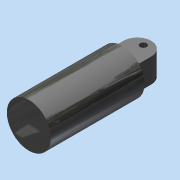
# Autodesk Inventor part: AntennaBase
Saved by Autodesk Inventor 2011 SP1 (Build 150282100, 282)
## iProperties
Created: 2011-08-14
Part Number: AntennaBase
Document SubType Name: Modeling
Designer: dgitz
Density: 1 g/cm^3
Author: dgitz
Autodesk Inventor part; units mm, degrees
ref_plane "YZ Plane" through (0, 0, 0) normal (1, 0, 0) x (0, 1, 0)
ref_plane "XZ Plane" through (0, 0, 0) normal (0, 1, 0) x (-1, 0, 0)
ref_plane "XY Plane" through (0, 0, 0) normal (0, 0, 1) x (1, 0, 0)
sketch "Sketch1" plane through (0, 0, 0) normal (0, 0, 1) x (1, 0, 0)
  point P0 (0, 0)
sketch "Sketch2" plane through (0, 0, 0) normal (0, 0, 1) x (1, 0, 0)
  circle A0 centre (0, 0) radius 5.08
  dimension "d0" = 10.16
  constraints: 1 centre point, 1 coincident
  measures "d0" diameter of A0
extrude "Extrusion1" add sketch "Sketch2" along normal blind 21.59
sketch "Sketch3" plane through (0, 0, 0) normal (0, 1, 0) x (-1, 0, 0)
  line L0 (0, -6.604) -> (0, -6.604)
  line L1 (3.175, -3.429) -> (3.175, 0)
  line L2 (3.175, 0) -> (-3.175, 0)
  line L3 (-3.175, 0) -> (-3.175, -3.429)
  circle A0 centre (0, -4.826) radius 0.762
  arc A1 (-3.175, -3.429) -> (0, -6.604) centre (0, -3.429) ccw
  arc A2 (0, -6.604) -> (3.175, -3.429) centre (0, -3.429) ccw
  point P0 (0, 0)
  dimension "d3" = 6.35
  dimension "d4" = 3.175
  dimension "d5" = 6.604
  dimension "d6" = 1.524
  dimension "d7" = 4.064
  dimension "d8" = 3.175
  constraints: 8 end point, 4 point on circle, 4 tangent, 3 centre point, 2 parallel, 1 concentric, 1 horizontal, 1 midpoint, 1 perpendicular
  measures "d3" distance between parallel lines of L1 L3
  measures "d4" distance from line of point (0, 0) L3
  measures "d5" distance between parallel lines of L2 L0
  measures "d6" diameter of A0
  measures "d7" distance edge to line of A0 L2
  measures "d8" radius of A1
extrude "Extrusion2" add sketch "Sketch3" along normal mid plane 5.588
body "Solid1"
